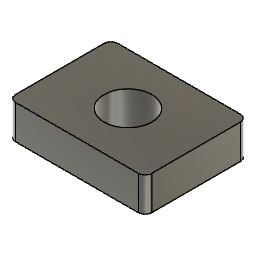
3D_Manufacturing_model (Autodesk Fusion 360 design; units mm, degrees)
Autodesk Fusion 360 part; units mm, degrees
sketch "Sketch1" plane through (0, 0, 0) normal (0, 0, 1) x (1, 0, 0)
  line L0 (-50, 37.5) -> (50, 37.5)
  line L1 (50, 37.5) -> (50, -37.5)
  line L2 (50, -37.5) -> (-50, -37.5)
  line L3 (-50, -37.5) -> (-50, 37.5)
  line L4 (-50, 37.5) -> (50, -37.5) construction
  line L5 (50, 37.5) -> (-50, -37.5) construction
  circle A0 centre (0, 0) radius 17.5
  dimension "d1" = 100
  dimension "d2" = 75
  dimension "d3" = 35
  constraint horizontal L0
  constraint perpendicular L0 L1
  constraint parallel L0 L2
  constraint parallel L1 L3
  constraint coincident L4 A0.centre
  constraint coincident L5 A0.centre
  constraint coincident A0.centre origin
  measures "d1" distance of L0.start L0.end
  measures "d2" distance of L0.start L2.end
  measures "d3" diameter of A0
extrude "Extrude1" add sketch "Sketch1" along normal blind 25
fillet "Fillet1" radius 5 4 edges at (50, -37.5, 12.5) (50, 37.5, 12.5) (-50, 37.5, 12.5) (-50, -37.5, 12.5)
